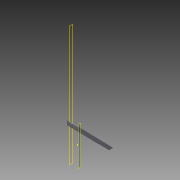
# Autodesk Inventor part: staircase
Saved by Autodesk Inventor 2015 (Build 190159000, 159)
## iProperties
Created: 2014-12-20
Part Number: staircase
Material: Generic
Document SubType Name: Modeling
Designer: jesse
Density: 1 g/cm^3
Appearance: Default
Author: jesse
Autodesk Inventor part; units mm, degrees
ref_plane "YZ Plane" through (0, 0, 0) normal (1, 0, 0) x (0, 1, 0)
ref_plane "XZ Plane" through (0, 0, 0) normal (0, 1, 0) x (-1, 0, 0)
ref_plane "XY Plane" through (0, 0, 0) normal (0, 0, 1) x (1, 0, 0)
ref_plane "Work Plane1" through (-1092.4793, 1301.7289, 0) normal (-1, 0, 0) x (0, 0, 1)
sketch "Sketch1" plane through (-1092.4793, 1301.7289, 0) normal (-1, 0, 0) x (0, 0, 1)
  line L0 (-203.2, -2770.4457) -> (-203.2, -2759.1173) projected
  line L1 (0, -2770.4457) -> (-203.2, -2770.4457) construction
  line L2 (0, 0) -> (0, -2770.4457) construction
  line L3 (0, 0) -> (-203.2, 0) construction
  line L4 (-203.2, -2759.1173) -> (-203.2, 0) construction
  line L5 (0, 0) -> (-2800.35, -2872.0457)
  line L6 (-2800.35, -2872.0457) -> (-2472.2016, -2872.0457)
  line L7 (-2472.2016, -2872.0457) -> (0, -336.5498)
  line L8 (0, -1046.0332) -> (-1780.4292, -2872.0457) construction
  line L9 (-1780.4292, -2872.0457) -> (-1656.265, -2872.0457) construction
  line L10 (-1656.265, -2872.0457) -> (0, -1173.3763) construction
  line L11 (0, -1173.3763) -> (0, -1046.0332) construction
  line L12 (0, 0) -> (0, -336.5498)
  point P0 (0, -1301.7289)
  dimension "d0" = 234.95
  dimension "d5" = 88.9
  dimension "d6" = 495.3
  constraints: 16 end point, 3 parallel, 3 point on line, 2 horizontal, 1 collinear, 1 other
  measures "d0" distance between parallel lines of L7 L5
  measures "d5" distance between parallel lines of L10 L8
  measures "d6" distance between parallel lines of L7 L8
extrude "Extrusion1" add sketch "Sketch1" along normal blind 38.1
ref_plane "Work Plane2" through (-1989.2009, -1457.3884, -438.15) normal (1, 0, 0) x (0, 0, -1)
sketch "Sketch2" plane through (-1989.2009, -1457.3884, -438.15) normal (1, 0, 0) x (0, 0, -1)
  line L0 (-438.15, 2759.1173) -> (2362.2, -112.9284) projected
  line L1 (2362.2, -112.9284) -> (2034.0516, -112.9284) projected
  line L2 (2034.0516, -112.9284) -> (-438.15, 2422.5675) projected
  line L3 (-438.15, 2422.5675) -> (-438.15, 2759.1173) projected
  point P0 (-438.15, 1457.3884)
extrude "Extrusion2" add sketch "Sketch2" along normal blind 38.1
sketch "Sketch4" plane through (-1130.5793, 1301.7289, 0) normal (-1, 0, 0) x (0, 0, 1)
  point P0 (0, -1301.7289)
sketch "Sketch5" plane through (-1130.5793, 1301.7289, 0) normal (-1, 0, 0) x (0, 0, 1)
  line L0 (-2800.35, -2872.0457) -> (-2472.2016, -2872.0457) projected
  line L1 (0, 0) -> (-2800.35, -2872.0457) projected
  line L2 (-2539.3566, -2872.0457) -> (-2577.4566, -2872.0457)
  line L3 (-2577.4566, -2872.0457) -> (-2577.4566, -2643.4457)
  line L4 (-2577.4566, -2643.4457) -> (-2539.3566, -2643.4457)
  line L5 (-2539.3566, -2643.4457) -> (-2539.3566, -2872.0457)
  point P0 (0, -1301.7289)
  dimension "d7" = 228.6
  dimension "d8" = 38.1
  constraints: 8 end point, 2 parallel, 2 point on line, 1 horizontal, 1 perpendicular
  measures "d7" distance of L4.end L2.start
  measures "d8" distance of L3.end L4.end
extrude "Extrusion3" add sketch "Sketch5" along normal up to surface (820.5216 mm away) contours L3 L4 L5 L0
pattern_linear "Rectangular Pattern1" count 16 spacing 234.95 along (0, 0.715987, 0.6981136) of "Extrusion3"
body "Solid1"
